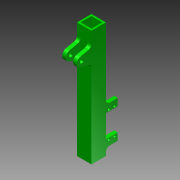
# Autodesk Inventor part: TableMount-Base
Saved by Autodesk Inventor 2012 (Build 160160000, 160)
## iProperties
Created: 2013-07-16
Part Number: TableMount-Base
Material: ABS Plastic
Document SubType Name: Modeling
Designer: joe_000
Density: 1.06 g/cm^3
Mass: 70.6052 g
Surface Area: 410 cm^2
Volume: 66.6086 cm^3
PivotOpeningWidth: 0.500 in
PivotHeight: 0.750 in
PivotAngle: 102.50 deg
PivotScrewDiameter: 0.250 in
PivotWidth: 1.000 in
Author: joe_000
Autodesk Inventor part; units mm, degrees
ref_plane "YZ Plane" through (0, 0, 0) normal (1, 0, 0) x (0, 1, 0)
ref_plane "XZ Plane" through (0, 0, 0) normal (0, 1, 0) x (-1, 0, 0)
ref_plane "XY Plane" through (0, 0, 0) normal (0, 0, 1) x (1, 0, 0)
sketch "Sketch2" plane through (0, 0, 0) normal (0, 1, 0) x (-1, 0, 0)
  line L0 (0, 0) -> (-25.4, 0)
  line L1 (-25.4, 0) -> (-25.4, -25.4)
  line L2 (-25.4, -25.4) -> (0, -25.4)
  line L3 (0, -25.4) -> (0, 0)
  line L4 (-3.175, -22.225) -> (-22.225, -22.225)
  line L5 (-22.225, -22.225) -> (-22.225, -3.175)
  line L6 (-22.225, -3.175) -> (-3.175, -3.175)
  line L7 (-3.175, -3.175) -> (-3.175, -22.225)
  dimension "d4" = 3.175
  dimension "d5" = 3.175
  dimension "d6" = 19.05
  dimension "d7" = 19.05
  dimension "d8" = 3.175
  dimension "d9" = 3.175
  constraints: 16 end point, 4 parallel, 2 horizontal, 2 perpendicular
  measures "d4" distance between parallel lines of L2 L4
  measures "d5" distance between parallel lines of L1 L5
  measures "d6" distance of L5.end L6.end
  measures "d7" distance of L6.end L4.start
  measures "d8" distance between parallel lines of L3 L7
  measures "d9" distance between parallel lines of L0 L6
extrude "Extrusion1" add sketch "Sketch2" along normal blind 203.2
sketch "Sketch3" plane through (25.4, 0, 0) normal (1, 0, 0) x (0, 0, -1)
  line L0 (0, 0) -> (25.4, 0) projected
  line L1 (25.4, 0) -> (25.4, 203.2) projected
  line L2 (25.4, 12.7) -> (46.2, 12.7)
  line L3 (46.2, 12.7) -> (46.2, 25.4)
  line L4 (46.2, 25.4) -> (25.4, 25.4)
  line L5 (25.4, 25.4) -> (25.4, 12.7)
  line L6 (25.4, 65.2112) -> (46.2, 65.2112)
  line L7 (46.2, 65.2112) -> (46.2, 77.9112)
  line L8 (46.2, 77.9112) -> (25.4, 77.9112)
  line L9 (25.4, 77.9112) -> (25.4, 65.2112)
  dimension "d12" = 39.8112
  dimension "d13" = 20.8
  dimension "d14" = 12.7
  dimension "d15" = 12.7
  constraints: 16 end point, 4 parallel, 2 equal length, 2 horizontal, 2 perpendicular, 2 point on line
  measures "d12" distance between parallel lines of L4 L6
  measures "d13" distance of L7.end L8.end
  measures "d14" distance of L6.end L7.end
  measures "d15" distance between parallel lines of L2 L0
extrude "Extrusion2" add sketch "Sketch3" against normal blind 6.35
fillet "Fillet1" radius 6.35 4 edges at (22.225, 77.9112, -25.4) (22.225, 12.7, -25.4) (19.05, 19.05, -25.4) (19.05, 71.5612, -25.4)
sketch "Sketch4" plane through (25.4, 0, 0) normal (1, 0, 0) x (0, 0, -1)
  circle A0 centre (30.8, 68.2) radius 2
  circle A1 centre (40.8, 68.2) radius 2
  circle A2 centre (30.8, 22.4) radius 2
  circle A3 centre (40.8, 22.4) radius 2
  line L0 (46.2, 25.4) -> (25.4, 25.4) projected
  line L1 (25.4, 65.2112) -> (46.2, 65.2112) projected
  line L2 (46.2, 77.9112) -> (31.75, 77.9112) projected
  line L3 (25.4, 84.2612) -> (25.4, 203.2) projected
  line L4 (35.8, 65.2112) -> (35.8, 77.9112)
  dimension "d19" = 4
  dimension "d23" = 3
  dimension "d25" = 45.8
  dimension "d26" = 5
  dimension "d28" = 10
  constraints: 4 centre point, 3 equal radius, 2 end point, 2 horizontal alignment, 2 vertical alignment, 1 midpoint, 1 parallel, 1 point on line
  measures "d19" diameter of A0
  measures "d23" distance from line of L0 A3.centre
  measures "d25" distance of A1.centre A3.centre
  measures "d26" distance from line of L4 A0.centre
  measures "d28" distance of A1.centre A0.centre
extrude "Extrusion3" cut sketch "Sketch4" against normal through all
sketch "Sketch5" plane through (25.4, 0, 0) normal (1, 0, 0) x (0, 0, -1)
  line L0 (0, 33.4612) -> (0, 203.2)
  line L1 (0, 177.8) -> (-19.05, 173.5767)
  line L2 (0, 152.4) -> (-19.05, 156.6233)
  arc A0 (-19.05, 173.5767) -> (-19.05, 156.6233) centre (-17.1708, 165.1) ccw
  circle A1 centre (-17.1708, 165.1) radius 3.175
  point P0 (0, -50.8)
  dimension "d29" = 25
  dimension "PivotWidth" = 25.4
  dimension "PivotHeight" = 19.05
  dimension "PivotAngle" = 102.5
  dimension "d33" = 203.2
  dimension "PivotScrewDiameter" = 6.35
  constraints: 6 end point, 2 centre point, 2 point on circle, 2 point on line, 1 coincident, 1 tangent, 1 vertical alignment
  measures "d29" angle of L2 L1
  measures "PivotWidth" distance of L2.start L1.start
  measures "PivotHeight" horizontal distance of L2.start L2.end
  measures "PivotAngle" angle of L0 L1
  measures "d33" distance of point (0, -50.8) L2.start
  measures "PivotScrewDiameter" diameter of A1
extrude "Extrusion4" add sketch "Sketch5" against normal blind 6.35
ref_plane "Work Plane1" through (12.7, 0, 0) normal (1, 0, 0) x (0, 0, -1)
mirror "Mirror1" about plane through (12.7, 0, 0) normal (1, 0, 0) of "Extrusion4"
sketch "Sketch6" plane through (25.4, 177.8, 0) normal (0, 0.976296, 0.2164396) x (1, 0, 0)
  line L0 (-19.05, 0) -> (-19.05, -19.5125) projected
  line L1 (-25.4, 0) -> (-25.4, -19.5125) projected
  line L2 (-25.4, 0) -> (-25.4, -19.5125) projected
  line L3 (-25.4, -19.5125) -> (-19.05, -19.5125) projected
  line L4 (-6.35, 0) -> (-6.35, -19.5125) projected
  point P0 (0, 6.35)
  point P1 (0, 0)
  point P2 (-25.4, -38.483)
  point P3 (0, 19.05)
  point P4 (6.35, -24.7979)
  point P5 (0, -24.7979)
  dimension "PivotOpeningWidth" = 12.7
  constraints: 4 other
fillet "Fillet3" radius 6.35 4 edges at (22.225, 177.8, 0) (3.175, 177.8, 0) (3.175, 152.4, 0) (22.225, 152.4, 0)
sketch "Sketch7" plane through (25.4, 0, -25.4) normal (0, 0, -1) x (-1, 0, 0)
  line L0 (25.4, 203.2) -> (0, 203.2) projected
  line L1 (12.7, 6.35) -> (12.7, 25.4) projected
  circle A0 centre (12.7, 177.8) radius 3.175
  line L2 (12.7, 203.2) -> (12.7, 165.4188)
  dimension "d40" = 6.35
  dimension "d41" = 25.4
  constraints: 2 end point, 1 centre point, 1 collinear, 1 midpoint, 1 point on line
  measures "d40" diameter of A0
  measures "d41" distance from line of L0 A0.centre
extrude "Extrusion5" cut sketch "Sketch7" against normal blind 12.7
equation "\"d4\" = MastSupportWallThickness"
equation "\"d5\" = MastSupportWallThickness"
equation "\"d6\" = MastWidth"
equation "\"d7\" = MastWidth"
equation "\"d8\" = MastSupportWallThickness"
equation "\"d9\" = MastSupportWallThickness"
equation "\"d12\" = ServoLength + ServoTolerance"
equation "\"d13\" = ServoWidth + ServoTolerance"
equation "\"d23\" = ServoScrewOffsetFromSide - 0.5 * ServoTolerance"
equation "\"d25\" = ServoScrewSpacingLength"
equation "\"d26\" = 0.5 * ServerScrewSpacing"
equation "\"d28\" = ServerScrewSpacing"
equation "\"MastSupportWallThickness\" = 3.175"
equation "\"ServoLength\" = 38.8112"
equation "\"ServoWidth\" = 19.8"
equation "\"ServerScrewSpacing\" = 10"
equation "\"ServoScrewOffsetFromSide\" = 3.5"
equation "\"ServoScrewSpacingLength\" = 45.8"
equation "\"ServoTolerance\" = 1"
equation "\"MastWidth\" = 19.05"
body "Solid1"
